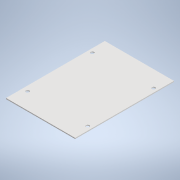
# Autodesk Inventor part: chasis
Saved by Autodesk Inventor 2020 (Build 240168000, 168)
## iProperties
Created: 2020-12-22
Part Number: chasis
Material: Generic
Document SubType Name: Modeling
Designer: Vikki
Density: 1 g/cm^3
Appearance: Default
Author: Vikki
Autodesk Inventor part; units mm, degrees
ref_plane "YZ Plane" through (0, 0, 0) normal (1, 0, 0) x (0, 1, 0)
ref_plane "XZ Plane" through (0, 0, 0) normal (0, 1, 0) x (-1, 0, 0)
ref_plane "XY Plane" through (0, 0, 0) normal (0, 0, 1) x (1, 0, 0)
sketch "Sketch1" plane through (0, 0, 0) normal (0, 1, 0) x (-1, 0, 0)
  line L0 (-105, 150) -> (105, 150)
  line L1 (105, 150) -> (105, -150)
  line L2 (105, -150) -> (-105, -150)
  line L3 (-105, -150) -> (-105, 150)
  line L4 (-105, 150) -> (105, -150) construction
  line L5 (105, 150) -> (-105, -150) construction
  circle A0 centre (-55, 130) radius 5
  circle A1 centre (55, 130) radius 5
  circle A2 centre (55, -100) radius 5
  circle A3 centre (-55, -100) radius 5
  point P0 (0, 0)
  dimension "d0" = 210
  dimension "d1" = 300
  dimension "d2" = 50
  dimension "d3" = 10
  dimension "d4" = 20
  dimension "d5" = 50
  dimension "d6" = 20
  dimension "d7" = 50
  dimension "d8" = 50
  dimension "d9" = 50
  dimension "d10" = 50
  constraints: 12 end point, 4 centre point, 3 equal radius, 2 midpoint, 2 parallel, 1 horizontal, 1 perpendicular
  measures "d0" distance of L1.end L2.end
  measures "d1" distance of L0.end L1.end
  measures "d2" distance from line of L3 A0.centre
  measures "d3" diameter of A0
  measures "d4" distance from line of L0 A0.centre
  measures "d5" distance from line of A1.centre L1
  measures "d6" distance from line of L0 A1.centre
  measures "d7" horizontal distance of L1.end A2.centre
  measures "d8" distance from line of L1 A2.centre
  measures "d9" distance from line of L2 A3.centre
  measures "d10" distance from line of L3 A3.centre
extrude "Extrusion1" add sketch "Sketch1" along normal blind 3
sketch "Sketch2" plane through (0, 0, 0) normal (0, -1, 0) x (1, 0, 0)
  circle A0 centre (-55, 130) radius 5 projected
  circle A1 centre (-55, 130) radius 11
  circle A2 centre (55, 130) radius 5 projected
  circle A3 centre (55, 130) radius 11
  point P0 (0, 0)
  dimension "d13" = 22
  constraints: 2 centre point, 2 coincident, 1 equal radius
  measures "d13" diameter of A3
extrude "Extrusion2" cut sketch "Sketch2" against normal blind 1
ref_plane "Work Plane1" through (0, 0, 150) normal (1, 0, 0) x (0, 0, -1)
equation "\"d5\" = d2"
equation "\"d8\" = d2"
equation "\"d10\" = d2"
body "Solid1"
